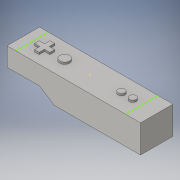
# Autodesk Inventor part: wiimote
Saved by Autodesk Inventor 2016 SP1 (Build 200210100, 210)
## iProperties
Created: 2016-05-01
Part Number: wiimote
Material: Generic
Document SubType Name: Modeling
Designer: Wes
Density: 1 g/cm^3
Appearance: Default
Author: Wes
Autodesk Inventor part; units mm, degrees
ref_plane "YZ Plane" through (0, 0, 0) normal (1, 0, 0) x (0, 1, 0)
ref_plane "XZ Plane" through (0, 0, 0) normal (0, 1, 0) x (-1, 0, 0)
ref_plane "XY Plane" through (0, 0, 0) normal (0, 0, 1) x (1, 0, 0)
sketch "Sketch1" plane through (0, 0, 0) normal (0, 1, 0) x (-1, 0, 0)
  line L0 (-74.6125, -18.1483) -> (74.6125, -18.1483)
  line L1 (74.6125, -18.1483) -> (74.6125, 18.1483)
  line L2 (74.6125, 18.1483) -> (-74.6125, 18.1483)
  line L3 (-74.6125, 18.1483) -> (-74.6125, -18.1483)
  line L4 (74.6125, -18.1483) -> (37.8079, -18.1483)
  line L5 (37.8079, -18.1483) -> (37.8079, 18.1483)
  line L6 (37.8079, 18.1483) -> (74.6125, 18.1483)
  line L7 (74.6125, 18.1483) -> (74.6125, -18.1483)
  line L8 (21.7678, 18.1483) -> (-74.6125, 18.1483)
  line L9 (-74.6125, 18.1483) -> (-74.6125, -18.1483)
  line L10 (-74.6125, -18.1483) -> (21.7678, -18.1483)
  line L11 (21.7678, -18.1483) -> (21.7678, 18.1483)
  line L12 (59.5566, 2.667) -> (42.1449, 2.667)
  line L13 (42.1449, 2.667) -> (42.1449, -2.667)
  line L14 (42.1449, -2.667) -> (59.5566, -2.667)
  line L15 (59.5566, -2.667) -> (59.5566, 2.667)
  line L16 (53.5178, 8.7058) -> (48.1838, 8.7058)
  line L17 (48.1838, 8.7058) -> (48.1838, -8.7058)
  line L18 (48.1838, -8.7058) -> (53.5178, -8.7058)
  line L19 (53.5178, -8.7058) -> (53.5178, 8.7058)
  circle A0 centre (-47.8282, 0) radius 3.7846
  circle A1 centre (-35.1917, 0) radius 3.7846
  circle A2 centre (28.2448, 0) radius 5.4546
  point P0 (0, 0)
  point P1 (50.8508, 0)
  dimension "d0" = 149.225
  dimension "d1" = 36.2966
  dimension "d2" = 36.8046
  dimension "d11" = 17.4117
  dimension "d12" = 5.334
  dimension "d13" = 5.334
  dimension "d14" = 17.4117
  dimension "d15" = 7.5692
  dimension "d16" = 7.5692
  dimension "d17" = 10.9093
  constraints: 40 end point, 10 parallel, 5 horizontal, 5 perpendicular, 3 centre point, 2 point on line
  measures "d0" distance of L2.end L1.end
  measures "d1" distance of L1.end L0.end
  measures "d2" distance of L5.end L6.end
  measures "d11" distance of L14.end L13.end
  measures "d12" distance of L13.end L12.end
  measures "d13" distance of L18.end L17.end
  measures "d14" distance of L17.end L16.end
  measures "d15" diameter of A0
  measures "d16" diameter of A1
  measures "d17" diameter of A2
extrude "Battery" add sketch "Sketch1" against normal blind 31.2166 contours L3 L2 L11 L0 | A0 | A1
extrude "Sensor" add sketch "Sketch1" against normal blind 20.7391 contours L5 L2 L1 L0 | L15 L14 L19 L12 | L19 L14 L17 L12 | L12 L17 L16 L19 | L17 L14 L13 L12 | L19 L18 L17 L14
loft "Loft1" add section 1 edges at (-37.8079, 0, 0) (-37.8079, -10.3696, 18.1483) (-37.8079, -20.7391, 0) (-37.8079, -10.3696, -18.1483) section 2 edges at (-21.7678, 0, 0) (-21.7678, -15.6083, -18.1483) (-21.7678, -31.2166, 0) (-21.7678, -15.6083, 18.1483)
extrude "1 Button" add sketch "Sketch1" along normal blind 2.032 contours A1
extrude "2 Button" add sketch "Sketch1" along normal blind 2.032 contours A0
extrude "A Button" add sketch "Sketch1" along normal blind 2.032 contours A2
extrude "D-Pad" add sketch "Sketch1" along normal blind 2.032 contours L15 L14 L19 L12 | L19 L14 L17 L12 | L12 L17 L16 L19 | L17 L14 L13 L12 | L19 L18 L17 L14
sketch "Sketch2" plane through (0, 0, 0) normal (0, 1, 0) x (1, 0, 0)
  line L0 (57.8104, -18.1483) -> (57.8104, 18.1483)
  line L1 (-64.8843, -18.1483) -> (-64.8843, 18.1483)
  point P0 (0, 0)
  constraints: 4 end point, 1 vertical
body "Solid1"
